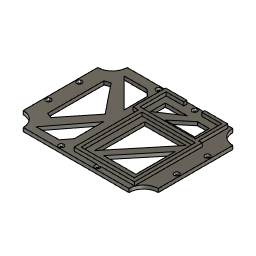
ipbox_floor v2 (Autodesk Fusion 360 design; units mm, degrees)
Autodesk Fusion 360 part; units mm, degrees
sketch "Sketch1" plane through (0, 0, 0) normal (0, 0, 1) x (1, 0, 0)
  line L0 (-75, 75) -> (155, 75)
  line L1 (155, 75) -> (155, -102)
  line L2 (155, -102) -> (-75, -102)
  line L3 (-75, -102) -> (-75, 75)
  circle A0 centre (-75, 75) radius 25
  circle A1 centre (155, 75) radius 25
  circle A2 centre (155, -102) radius 25
  circle A3 centre (-75, -102) radius 25
  line L4 (-75, 75) -> (155, -102)
  line L5 (155, 75) -> (-75, -102)
  line L6 (70.75, -39.75) -> (9.25, -39.75)
  line L7 (9.25, -39.75) -> (9.25, 12.75)
  line L8 (9.25, 12.75) -> (70.75, 12.75)
  line L9 (70.75, 12.75) -> (70.75, -39.75)
  line L10 (70.75, -39.75) -> (9.25, 12.75) construction
  line L11 (9.25, -39.75) -> (70.75, 12.75) construction
  line L12 (9.25, 12.75) -> (9.25, -39.75)
  line L13 (9.25, -39.75) -> (-69.15, -39.75)
  line L14 (-69.15, -39.75) -> (-69.15, 12.75)
  line L15 (-69.15, 12.75) -> (9.25, 12.75)
  line L16 (70.75, 12.75) -> (70.75, -39.75)
  line L17 (70.75, -39.75) -> (149.15, -39.75)
  line L18 (149.15, -39.75) -> (149.15, 12.75)
  line L19 (149.15, 12.75) -> (70.75, 12.75)
  line L20 (9.25, 12.75) -> (70.75, 12.75)
  line L21 (70.75, 12.75) -> (70.75, 69.45)
  line L22 (70.75, 69.45) -> (9.25, 69.45)
  line L23 (9.25, 69.45) -> (9.25, 12.75)
  line L24 (9.25, -39.75) -> (70.75, -39.75)
  line L25 (70.75, -39.75) -> (70.75, -96.45)
  line L26 (70.75, -96.45) -> (9.25, -96.45)
  line L27 (9.25, -96.45) -> (9.25, -39.75)
  circle A4 centre (9.25, 69.45) radius 1.9
  circle A5 centre (70.75, 69.45) radius 1.9
  circle A6 centre (149.15, 12.75) radius 1.9
  circle A7 centre (149.15, -39.75) radius 1.9
  circle A8 centre (70.75, -96.45) radius 1.9
  circle A9 centre (9.25, -96.45) radius 1.9
  circle A10 centre (-69.15, -39.75) radius 1.9
  circle A11 centre (-69.15, 12.75) radius 1.9
  point P0 (40, -13.5)
  dimension "d1" = 230
  dimension "d2" = 177
  dimension "d3" = 50
  dimension "d4" = 50
  dimension "d5" = 50
  dimension "d6" = 50
  dimension "d7" = 61.5
  dimension "d8" = 52.5
  dimension "d9" = 78.4
  dimension "d10" = 78.4
  dimension "d11" = 56.7
  dimension "d12" = 56.7
  dimension "d13" = 3.8
  dimension "d14" = 3.8
  dimension "d15" = 3.8
  dimension "d16" = 3.8
  dimension "d17" = 3.8
  dimension "d18" = 3.8
  dimension "d19" = 3.8
  dimension "d20" = 3.8
  constraint horizontal L0
  constraint vertical L1
  constraint horizontal L2
  constraint vertical L3
  constraint coincident L0.start L3.end
  constraint coincident L0.end L1.start
  constraint coincident L1.end L2.start
  constraint coincident L2.end L3.start
  constraint horizontal L6
  constraint perpendicular L6 L7
  constraint parallel L6 L8
  constraint parallel L7 L9
  constraint coincident L10 P0
  constraint coincident L11 P0
  constraint midpoint L5 P0
  constraint perpendicular L12 L13
  constraint parallel L12 L14
  constraint parallel L13 L15
  constraint perpendicular L16 L17
  constraint parallel L16 L18
  constraint parallel L17 L19
  constraint perpendicular L20 L21
  constraint parallel L20 L22
  constraint parallel L21 L23
  constraint perpendicular L24 L25
  constraint parallel L24 L26
  constraint parallel L25 L27
  constraint coincident L22.end L23.start
  constraint coincident L21.end L22.start
  constraint coincident L18.end L19.start
  constraint coincident L17.end L18.start
  constraint coincident L25.end L26.start
  constraint coincident L26.end L27.start
  constraint coincident L13.end L14.start
  constraint coincident L14.end L15.start
  measures "d1" distance of L0.start L0.end
  measures "d2" distance of L0.start L2.end
  measures "d3" diameter of A0
  measures "d4" diameter of A1
  measures "d5" diameter of A2
  measures "d6" diameter of A3
  measures "d7" distance of L7.end L8.end
  measures "d8" distance of L6.end L7.end
  measures "d9" distance of L7.end L14.end
  measures "d10" distance of L8.end L18.end
  measures "d11" distance of L7.end L22.end
  measures "d12" distance of L6.end L26.end
  measures "d13" diameter of A4
  measures "d14" diameter of A5
  measures "d15" diameter of A6
  measures "d16" diameter of A7
  measures "d17" diameter of A8
  measures "d18" diameter of A9
  measures "d19" diameter of A10
  measures "d20" diameter of A11
extrude "Extrude5" add sketch "Sketch1" along normal blind 6 contours L0 A0 A1 L4 L5 L15 L19 L21 L22 L23 A4 A5 | L3 A0 A3 L4 L5 L13 L14 L15 A10 A11 | L4 L7 L12 L15 | L4 L5 L7 L12 L13 L14 L15 A10 A11 | L1 A1 A2 L4 L5 L17 L18 L19 A6 A7 | L2 A2 A3 L4 L5 L13 L17 L25 L26 L27 A8 A9 | L4 L5 L7 L8 L9 L12 L16 L20 | L4 L5 L7 L12 | L8 L20 L21 L22 L23 A4 A5 | L4 L5 L9 L16 L17 L18 L19 A6 A7 | L5 L9 L16 L19 | L5 L7 L12 L13 | L4 L5 L9 L16 | L4 L5 L6 L7 L9 L12 L16 L24 | L6 L24 L25 L26 L27 A8 A9 | L4 L9 L16 L17
sketch "Sketch4" plane through (0, 0, 6) normal (0, 0, 1) x (-1, 0, 0)
  circle A0 centre (69.15, 39.75) radius 1.9
  circle A1 centre (-70.75, 96.45) radius 1.9
  circle A2 centre (-9.25, -69.45) radius 1.9
  circle A3 centre (-149.15, 39.75) radius 1.9
  circle A4 centre (69.15, -12.75) radius 1.9
  circle A5 centre (-149.15, -12.75) radius 1.9
  circle A6 centre (-70.75, -69.45) radius 1.9
  circle A7 centre (-9.25, 96.45) radius 1.9
  line L0 (50, 102) -> (-130, 102)
  arc A8 (-155, 77) -> (-130, 102) centre (-155, 102) ccw
  line L1 (-155, 77) -> (-155, -50)
  arc A9 (-130, -75) -> (-155, -50) centre (-155, -75) ccw
  line L2 (-130, -75) -> (50, -75)
  arc A10 (75, -50) -> (50, -75) centre (75, -75) ccw
  line L3 (75, -50) -> (75, 77)
  arc A11 (50, 102) -> (75, 77) centre (75, 102) ccw
  line L4 (-125, 87.5) -> (-34.3, 87.5)
  line L5 (-34.3, 87.5) -> (-34.3, -16)
  line L6 (-34.3, -16) -> (-125, -16)
  line L7 (-125, -16) -> (-125, 87.5)
  line L8 (-34.3, -16) -> (-28.3, -16)
  line L9 (-28.3, -16) -> (-28.3, -22)
  line L10 (-28.3, -22) -> (-34.3, -22)
  line L11 (-34.3, -22) -> (-34.3, -16)
  line L12 (-125, 87.5) -> (-131, 87.5)
  line L13 (-131, 87.5) -> (-131, 93.5)
  line L14 (-131, 93.5) -> (-125, 93.5)
  line L15 (-125, 93.5) -> (-125, 87.5)
  line L16 (-28.3, -22) -> (-131, -22)
  line L17 (-131, -22) -> (-131, 93.5)
  line L18 (-131, 93.5) -> (-28.3, 93.5)
  line L19 (-28.3, 93.5) -> (-28.3, -22)
  line L20 (-119.51, -22) -> (-25.01, -22)
  line L21 (-25.01, -22) -> (-25.01, -66.5)
  line L22 (-25.01, -66.5) -> (-119.51, -66.5)
  line L23 (-119.51, -66.5) -> (-119.51, -22)
  line L24 (-25.01, -66.5) -> (-19.01, -66.5)
  line L25 (-19.01, -66.5) -> (-19.01, -71.5)
  line L26 (-19.01, -71.5) -> (-25.01, -71.5)
  line L27 (-25.01, -71.5) -> (-25.01, -66.5)
  line L28 (-19.01, -71.5) -> (-125, -71.5)
  line L29 (-125, -71.5) -> (-125, -16)
  line L30 (-125, -16) -> (-19.01, -16)
  line L31 (-19.01, -16) -> (-19.01, -71.5)
  line L32 (-55.2748, -71.5) -> (-85.643, -71.5)
  line L33 (-85.643, -71.5) -> (-85.643, -66.5)
  line L34 (-85.643, -66.5) -> (-55.2748, -66.5)
  line L35 (-55.2748, -66.5) -> (-55.2748, -71.5)
  dimension "d44" = 90.7
  dimension "d45" = 103.5
  dimension "d46" = 6
  dimension "d47" = 6
  dimension "d48" = 6
  dimension "d49" = 6
  dimension "d50" = 94.5
  dimension "d51" = 44.5
  dimension "d52" = 6
  dimension "d53" = 5
  constraint horizontal L4
  constraint vertical L5
  constraint horizontal L6
  constraint vertical L7
  constraint horizontal L8
  constraint vertical L9
  constraint horizontal L10
  constraint vertical L11
  constraint horizontal L12
  constraint vertical L13
  constraint horizontal L14
  constraint vertical L15
  constraint horizontal L16
  constraint vertical L17
  constraint horizontal L18
  constraint vertical L19
  constraint horizontal L20
  constraint vertical L21
  constraint horizontal L22
  constraint vertical L23
  constraint coincident L16 L20.start
  constraint horizontal L24
  constraint vertical L25
  constraint horizontal L26
  constraint vertical L27
  constraint horizontal L28
  constraint vertical L29
  constraint horizontal L30
  constraint vertical L31
  constraint horizontal L32
  constraint vertical L33
  constraint horizontal L34
  constraint vertical L35
  constraint coincident L22 L33.end
  constraint coincident L28 L32.start
  measures "d44" distance of L4.start L4.end
  measures "d45" distance of L4.start L6.end
  measures "d46" distance of L5.end L8.end
  measures "d47" distance of L5.end L10.end
  measures "d48" distance of L4.start L12.end
  measures "d49" distance of L4.start L14.end
  measures "d50" distance of L20.start L20.end
  measures "d51" distance of L20.start L22.end
  measures "d52" distance of L21.end L24.end
  measures "d53" distance of L21.end L26.end
extrude "Extrude6" add sketch "Sketch4" along normal blind 6 contours L4 L5 L8 L15 L18 L19 L30 | L7 L12 L16 L17 L29 | L12 L13 L14 L15 L17 L18 | L6 L11 L16 L20 L29 L30 | L8 L9 L10 L11 L16 L19 L20 L30 | L16 L22 L23 L28 L29 L33 | L9 L19 L20 L21 L24 L30 L31 | L24 L25 L26 L27 L28 L31 | L22 L27 L28 L35
sketch "Sketch5" plane through (0, 0, 6) normal (0, 0, 1) x (-1, 0, 0)
  line L0 (50, 102) -> (-130, 102)
  arc A0 (-155, 77) -> (-130, 102) centre (-155, 102) ccw
  line L1 (-155, 77) -> (-155, -50)
  arc A1 (-130, -75) -> (-155, -50) centre (-155, -75) ccw
  line L2 (-130, -75) -> (50, -75)
  arc A2 (75, -50) -> (50, -75) centre (75, -75) ccw
  line L3 (75, -50) -> (75, 77)
  arc A3 (50, 102) -> (75, 77) centre (75, 102) ccw
  circle A4 centre (-9.25, 96.45) radius 1.9
  circle A5 centre (-70.75, -69.45) radius 1.9
  circle A6 centre (-149.15, -12.75) radius 1.9
  circle A7 centre (69.15, -12.75) radius 1.9
  circle A8 centre (-149.15, 39.75) radius 1.9
  circle A9 centre (-9.25, -69.45) radius 1.9
  circle A10 centre (-70.75, 96.45) radius 1.9
  circle A11 centre (69.15, 39.75) radius 1.9
  line L4 (-85.643, -71.5) -> (-125, -71.5)
  line L5 (-125, -71.5) -> (-125, -22)
  line L6 (-125, -22) -> (-131, -22)
  line L7 (-131, -22) -> (-131, 93.5)
  line L8 (-131, 93.5) -> (-28.3, 93.5)
  line L9 (-28.3, 93.5) -> (-28.3, -16)
  line L10 (-28.3, -16) -> (-19.01, -16)
  line L11 (-19.01, -16) -> (-19.01, -71.5)
  line L12 (-19.01, -71.5) -> (-55.2748, -71.5)
  line L13 (-55.2748, -71.5) -> (-55.2748, -66.5)
  line L14 (-55.2748, -66.5) -> (-25.01, -66.5)
  line L15 (-25.01, -66.5) -> (-25.01, -22)
  line L16 (-25.01, -22) -> (-119.51, -22)
  line L17 (-119.51, -22) -> (-119.51, -66.5)
  line L18 (-119.51, -66.5) -> (-85.643, -66.5)
  line L19 (-85.643, -66.5) -> (-85.643, -71.5)
  line L20 (50, -50) -> (50, 75)
  line L21 (50, 75) -> (0, 12.5)
  line L22 (0, 12.5) -> (50, -50)
  line L23 (40, 90) -> (-10, 25)
  line L24 (-10, 25) -> (-10, 75)
  line L25 (-10, 75) -> (1.1591, 89.5069)
  line L26 (1.1591, 89.5069) -> (40, 90)
  line L27 (40, -60) -> (1.1591, -60)
  line L28 (1.1591, -60) -> (-10, -50)
  line L29 (-10, -50) -> (-10, -10)
  line L30 (-10, -10) -> (40, -60)
  line L31 (-45, 75) -> (-45, -10)
  line L32 (-45, -10) -> (-115, -10)
  line L33 (-115, -10) -> (-45, 75)
  line L34 (-60, 75) -> (-115, 8.2143)
  line L35 (-115, 8.2143) -> (-115, 75)
  line L36 (-115, 75) -> (-60, 75)
  line L37 (-35, -30) -> (-35, -55)
  line L38 (-35, -55) -> (-72.26, -55)
  line L39 (-72.26, -55) -> (-35, -30)
  line L40 (-60, -30) -> (-90, -55)
  line L41 (-90, -55) -> (-110, -55)
  line L42 (-110, -55) -> (-110, -30)
  line L43 (-110, -30) -> (-60, -30)
  constraint vertical L20
  constraint parallel L20 L24
  constraint parallel L23 L25
  constraint perpendicular L24 L27
  constraint perpendicular L27 L31
  constraint perpendicular L31 L32
  constraint parallel L33 L34
  constraint perpendicular L32 L35
  constraint perpendicular L35 L36
  constraint perpendicular L16 L37
  constraint perpendicular L37 L38
  constraint parallel L38 L41
  constraint perpendicular L41 L42
  constraint perpendicular L42 L43
extrude "Extrude7" cut sketch "Sketch5" against normal blind 30 contours L20 L21 L22 | L23 L24 L25 L26 | L27 L28 L29 L30 | L31 L32 L33 | L34 L35 L36 | L37 L38 L39 | L40 L41 L42 L43
chamfer "Chamfer2" distance 14.5 angle 45 1 edges at (-50, 50, 3)
chamfer "Chamfer3" distance 14.5 angle 45 1 edges at (-50, -75, 3)
chamfer "Chamfer4" distance 2.5 angle 45 8 edges at (-70.9214, 13.4371, 6) (68.9786, 70.1371, 6) (7.4786, 70.1371, 6) (147.3786, 13.4371, 6) (147.3786, -39.0629, 6) (68.9786, -95.7629, 6) (7.4786, -95.7629, 6) (-70.9214, -39.0629, 6)
